Autodesk Inventor part; units mm, degrees
(part 2 of 2)
sketch "Sketch10" plane through (0, 0, 3.75) normal (0, 0, 1) x (1, 0, 0)
  line L0 (-21, 11) -> (-21, -11) projected
  line L1 (-21, -11) -> (-15, -11) projected
  line L2 (-15, -11) -> (-15, 11) projected
  line L3 (-15, 11) -> (-21, 11) projected
  line L4 (-20, 10) -> (-16, 10) projected
  line L5 (-16, 10) -> (-16, -10) projected
  line L6 (-16, -10) -> (-20, -10) projected
  line L7 (-20, -10) -> (-20, 10) projected
  line L8 (6, 21) -> (-6, 21) projected
  line L9 (-6, 21) -> (-6, 15) projected
  line L10 (-6, 15) -> (6, 15) projected
  line L11 (6, 15) -> (6, 21) projected
  line L12 (-5.1733, 20) -> (5.0327, 20) projected
  line L13 (5.0327, 20) -> (5.0327, 16) projected
  line L14 (5.0327, 16) -> (-5.1733, 16) projected
  line L15 (-5.1733, 16) -> (-5.1733, 20) projected
  line L16 (18.5, -10) -> (18.5, 9) projected
  line L17 (18.5, 9) -> (16, 9) projected
  line L18 (16, 9) -> (16, -10) projected
  line L19 (16, -10) -> (18.5, -10) projected
  line L20 (17.6346, -9) -> (16.861, -9) projected
  line L21 (16.861, -9) -> (16.861, -8) projected
  line L22 (16.861, -8) -> (17.6346, -8) projected
  line L23 (17.6346, -8) -> (17.6346, -9) projected
  line L24 (17.6346, -7) -> (16.861, -7) projected
  line L25 (16.861, -7) -> (16.861, -6) projected
  line L26 (16.861, -6) -> (17.6346, -6) projected
  line L27 (17.6346, -6) -> (17.6346, -7) projected
  line L28 (17.6346, -5) -> (16.861, -5) projected
  line L29 (16.861, -5) -> (16.861, -4) projected
  line L30 (16.861, -4) -> (17.6346, -4) projected
  line L31 (17.6346, -4) -> (17.6346, -5) projected
  line L32 (17.6346, -3) -> (16.861, -3) projected
  line L33 (16.861, -3) -> (16.861, -2) projected
  line L34 (16.861, -2) -> (17.6346, -2) projected
  line L35 (17.6346, -2) -> (17.6346, -3) projected
  line L36 (17.6337, -1.0613) -> (16.8602, -1.0613) projected
  line L37 (16.8602, -1.0613) -> (16.8602, -0.0613) projected
  line L38 (16.8602, -0.0613) -> (17.6337, -0.0613) projected
  line L39 (17.6337, -0.0613) -> (17.6337, -1.0613) projected
  line L40 (17.6337, 1.1028) -> (16.8602, 1.1028) projected
  line L41 (16.8602, 1.1028) -> (16.8602, 2.1028) projected
  line L42 (16.8602, 2.1028) -> (17.6337, 2.1028) projected
  line L43 (17.6337, 2.1028) -> (17.6337, 1.1028) projected
  line L44 (17.6346, 3) -> (16.861, 3) projected
  line L45 (16.861, 3) -> (16.861, 4) projected
  line L46 (16.861, 4) -> (17.6346, 4) projected
  line L47 (17.6346, 4) -> (17.6346, 3) projected
  line L48 (17.6346, 5) -> (16.861, 5) projected
  line L49 (16.861, 5) -> (16.861, 6) projected
  line L50 (16.861, 6) -> (17.6346, 6) projected
  line L51 (17.6346, 6) -> (17.6346, 5) projected
  line L52 (16.861, 8) -> (17.6346, 8) projected
  line L53 (17.6346, 8) -> (17.6346, 7) projected
  line L54 (17.6346, 7) -> (16.861, 7) projected
  line L55 (16.861, 7) -> (16.861, 8) projected
  line L56 (-19, -3) -> (-19, -2.5) projected
  line L57 (-19, -2.5) -> (-18.3156, -2.5) projected
  line L58 (-18.3156, -2.5) -> (-18.3156, -3) projected
  line L59 (-18.3156, -3) -> (-19, -3) projected
  line L60 (-19, 1.4327) -> (-19, 1.9327) projected
  line L61 (-19, 1.9327) -> (-18.3156, 1.9327) projected
  line L62 (-18.3156, 1.9327) -> (-18.3156, 1.4327) projected
  line L63 (-18.3156, 1.4327) -> (-19, 1.4327) projected
  line L64 (-19, 8) -> (-19, 8.5) projected
  line L65 (-19, 8.5) -> (-18.3156, 8.5) projected
  line L66 (-18.3156, 8.5) -> (-18.3156, 8) projected
  line L67 (-18.3156, 8) -> (-19, 8) projected
  line L68 (-20, 10) -> (-20, -10) projected
  line L69 (-20, -10) -> (-16, -10) projected
  line L70 (-16, -10) -> (-16, 10) projected
  line L71 (-16, 10) -> (-20, 10) projected
  line L72 (-19, -6) -> (-19, -5.5) projected
  line L73 (-19, -5.5) -> (-18.3156, -5.5) projected
  line L74 (-18.3156, -5.5) -> (-18.3156, -6) projected
  line L75 (-18.3156, -6) -> (-19, -6) projected
  line L76 (-19, 4.8259) -> (-19, 5.3259) projected
  line L77 (-19, 5.3259) -> (-18.3156, 5.3259) projected
  line L78 (-18.3156, 5.3259) -> (-18.3156, 4.8259) projected
  line L79 (-18.3156, 4.8259) -> (-19, 4.8259) projected
  line L80 (-19, -8.4464) -> (-19, -7.9464) projected
  line L81 (-19, -7.9464) -> (-18.3156, -7.9464) projected
  line L82 (-18.3156, -7.9464) -> (-18.3156, -8.4464) projected
  line L83 (-18.3156, -8.4464) -> (-19, -8.4464) projected
  line L84 (-5.1733, 20) -> (-5.1733, 16) projected
  line L85 (-5.1733, 16) -> (5.0327, 16) projected
  line L86 (5.0327, 16) -> (5.0327, 20) projected
  line L87 (5.0327, 20) -> (-5.1733, 20) projected
  line L88 (1.2968, 18.5) -> (1.2968, 19) projected
  line L89 (1.2968, 19) -> (2.1134, 19) projected
  line L90 (2.1134, 19) -> (2.1134, 18.5) projected
  line L91 (2.1134, 18.5) -> (1.2968, 18.5) projected
  line L92 (-4.3467, 18.5) -> (-4.3467, 19) projected
  line L93 (-4.3467, 19) -> (-3.5998, 19) projected
  line L94 (-3.5998, 19) -> (-3.5998, 18.5) projected
  line L95 (-3.5998, 18.5) -> (-4.3467, 18.5) projected
  line L96 (3.6544, 19) -> (4.5488, 19) projected
  line L97 (4.5488, 19) -> (4.5488, 18.5) projected
  line L98 (4.5488, 18.5) -> (3.6544, 18.5) projected
  line L99 (3.6544, 18.5) -> (3.6544, 19) projected
  line L100 (-1.5055, 18.5) -> (-1.5055, 19) projected
  line L101 (-1.5055, 19) -> (-0.7289, 19) projected
  line L102 (-0.7289, 19) -> (-0.7289, 18.5) projected
  line L103 (-0.7289, 18.5) -> (-1.5055, 18.5) projected
  point P0 (0, 0)
extrude "Extrusion10" add sketch "Sketch10" along normal blind 5.5
sketch "Sketch11" plane through (-16, 21, 0) normal (0, 1, 0) x (1, 0, 0)
  line L0 (10, -1.25) -> (10, -9.25) projected
  line L1 (22, -9.25) -> (10, -9.25) projected
  line L2 (22, -1.25) -> (22, -9.25) projected
  line L3 (22, -1.25) -> (22, -9.25) projected
  line L4 (10, -1.25) -> (22, -1.25)
  point P0 (16, 0)
  constraints: 2 end point, 1 perpendicular
extrude "Extrusion11" add sketch "Sketch11" along normal blind 0.005
sketch "Sketch12" plane through (21, -16, 0) normal (1, 0, 0) x (0, 0, -1)
  line L0 (-2.75, 24) -> (-2.75, 7) projected
  line L1 (-1.25, 7) -> (-2.75, 7) projected
  line L2 (-1.25, 24) -> (-2.75, 24) projected
  line L3 (-1.25, 24) -> (-1.25, 7)
  point P0 (0, 16)
  constraints: 2 end point
extrude "Extrusion12" add sketch "Sketch12" along normal blind 0.005
sketch "Sketch13" plane through (-21, -16, 0) normal (-1, 0, 0) x (0, 0, 1)
  line L0 (1.25, 5) -> (9.25, 5) projected
  line L1 (9.25, 27) -> (9.25, 5) projected
  line L2 (1.25, 27) -> (9.25, 27) projected
  line L3 (1.25, 27) -> (1.25, 5) projected
  line L4 (1.25, 27) -> (1.25, 5)
  point P0 (0, 16)
  constraints: 2 end point
extrude "Extrusion13" add sketch "Sketch13" along normal blind 0.005
sketch "Sketch14" plane through (0, 0, 1.25) normal (0, 0, 1) x (1, 0, 0)
  line L0 (6, -8.4464) -> (6, -10) projected
  line L1 (-8, 0) -> (-8, -7) projected
  line L2 (-13, -7) -> (-13, 0) projected
  line L3 (11, 2.5) -> (2.5, 2.5) projected
  line L4 (3.1309, 2.5) -> (4, 2.5)
  line L5 (4, 2.5) -> (4, 2)
  line L6 (4, 2) -> (3.1309, 2)
  line L7 (3.1309, 2) -> (3.1309, 2.5)
  line L8 (5.0085, 2.5) -> (5.8776, 2.5)
  line L9 (5.8776, 2.5) -> (5.8776, 2)
  line L10 (5.8776, 2) -> (5.0085, 2)
  line L11 (5.0085, 2) -> (5.0085, 2.5)
  line L12 (7.1309, 2.5) -> (8, 2.5)
  line L13 (8, 2.5) -> (8, 2)
  line L14 (8, 2) -> (7.1309, 2)
  line L15 (7.1309, 2) -> (7.1309, 2.5)
  line L16 (9.1309, 2.5) -> (10, 2.5)
  line L17 (10, 2.5) -> (10, 2)
  line L18 (10, 2) -> (9.1309, 2)
  line L19 (9.1309, 2) -> (9.1309, 2.5)
  line L20 (3.1309, 5.2581) -> (4, 5.2581)
  line L21 (4, 5.2581) -> (4, 4.7581)
  line L22 (4, 4.7581) -> (3.1309, 4.7581)
  line L23 (3.1309, 4.7581) -> (3.1309, 5.2581)
  line L24 (5.0085, 5.2581) -> (5.8776, 5.2581)
  line L25 (5.8776, 5.2581) -> (5.8776, 4.7581)
  line L26 (5.8776, 4.7581) -> (5.0085, 4.7581)
  line L27 (5.0085, 4.7581) -> (5.0085, 5.2581)
  line L28 (7.1309, 5.2581) -> (8, 5.2581)
  line L29 (8, 5.2581) -> (8, 4.7581)
  line L30 (8, 4.7581) -> (7.1309, 4.7581)
  line L31 (7.1309, 4.7581) -> (7.1309, 5.2581)
  line L32 (9.1309, 5.2581) -> (10, 5.2581)
  line L33 (10, 5.2581) -> (10, 4.7581)
  line L34 (10, 4.7581) -> (9.1309, 4.7581)
  line L35 (9.1309, 4.7581) -> (9.1309, 5.2581)
  line L36 (-13, -6.1309) -> (-13, -7)
  line L37 (-13, -7) -> (-13.5, -7)
  line L38 (-13.5, -7) -> (-13.5, -6.1309)
  line L39 (-13.5, -6.1309) -> (-13, -6.1309)
  line L40 (-13, -4.1309) -> (-13, -5)
  line L41 (-13, -5) -> (-13.5, -5)
  line L42 (-13.5, -5) -> (-13.5, -4.1309)
  line L43 (-13.5, -4.1309) -> (-13, -4.1309)
  line L44 (-13.5, -2.8776) -> (-13.5, -2.0085)
  line L45 (-13, -2.0085) -> (-13, -2.8776)
  line L46 (-13, -2.8776) -> (-13.5, -2.8776)
  line L47 (-13.5, -2.0085) -> (-13, -2.0085)
  line L48 (-13, -0.1309) -> (-13, -1)
  line L49 (-13, -1) -> (-13.5, -1)
  line L50 (-13.5, -1) -> (-13.5, -0.1309)
  line L51 (-13.5, -0.1309) -> (-13, -0.1309)
  line L52 (-14.5, 7.4915) -> (-14, 7.4915)
  line L53 (-7.5, -6.1309) -> (-7.5, -7)
  line L54 (-7.5, -7) -> (-8, -7)
  line L55 (-8, -7) -> (-8, -6.1309)
  line L56 (-8, -6.1309) -> (-7.5, -6.1309)
  line L57 (-7.5, -4.1309) -> (-7.5, -5)
  line L58 (-7.5, -5) -> (-8, -5)
  line L59 (-8, -5) -> (-8, -4.1309)
  line L60 (-8, -4.1309) -> (-7.5, -4.1309)
  line L61 (-8, -2.8776) -> (-8, -2.0085)
  line L62 (-7.5, -2.0085) -> (-7.5, -2.8776)
  line L63 (-7.5, -2.8776) -> (-8, -2.8776)
  line L64 (-8, -2.0085) -> (-7.5, -2.0085)
  line L65 (-7.5, -0.1309) -> (-7.5, -1)
  line L66 (-7.5, -1) -> (-8, -1)
  line L67 (-8, -1) -> (-8, -0.1309)
  line L68 (-8, -0.1309) -> (-7.5, -0.1309)
  line L69 (-14.5, 3.5) -> (-14.5, 4.3691)
  line L70 (-14.5, 4.3691) -> (-14, 4.3691)
  line L71 (-14, 3.5) -> (-14.5, 3.5)
  line L72 (-14, 4.3691) -> (-14, 3.5)
  line L73 (-14, 5.6224) -> (-14.5, 5.6224)
  line L74 (-14, 6.4915) -> (-14, 5.6224)
  line L75 (-14.5, 8.3691) -> (-14, 8.3691)
  line L76 (-14.5, 7.5) -> (-14.5, 8.3691)
  line L77 (-14, 8.3691) -> (-14, 7.5)
  line L78 (-14, 7.5) -> (-14.5, 7.5)
  line L79 (-14.5, 6.4915) -> (-14, 6.4915)
  line L80 (-14.5, 5.6224) -> (-14.5, 6.4915)
  line L81 (-11.9931, 3.557) -> (-11.9931, 4.426)
  line L82 (-11.9931, 4.426) -> (-11.4931, 4.426)
  line L83 (-11.4931, 3.557) -> (-11.9931, 3.557)
  line L84 (-11.4931, 4.426) -> (-11.4931, 3.557)
  line L85 (-11.4931, 5.6794) -> (-11.9931, 5.6794)
  line L86 (-11.4931, 6.5484) -> (-11.4931, 5.6794)
  line L87 (-11.9931, 8.426) -> (-11.4931, 8.426)
  line L88 (-11.9931, 7.557) -> (-11.9931, 8.426)
  line L89 (-11.4931, 8.426) -> (-11.4931, 7.557)
  line L90 (-11.4931, 7.557) -> (-11.9931, 7.557)
  line L91 (-11.9931, 6.5484) -> (-11.4931, 6.5484)
  line L92 (-11.9931, 5.6794) -> (-11.9931, 6.5484)
  line L93 (-14, 4.3691) -> (-14, 3.5)
  line L94 (-14, 8.3691) -> (-14, 7.4915)
  line L95 (-14, 6.4915) -> (-14, 5.6224)
  line L96 (1.713, -11.4558) -> (3.1309, -11.4558) projected
  line L97 (3.1309, -11.4558) -> (3.1309, -7) projected
  line L98 (3.1309, -7) -> (1.713, -7) projected
  line L99 (1.713, -7) -> (1.713, -11.4558) projected
  line L100 (6.25, -11.4558) -> (8, -11.4558) projected
  line L101 (8, -11.4558) -> (8, -7) projected
  line L102 (8, -7) -> (6.25, -7) projected
  line L103 (6.25, -7) -> (6.25, -11.4558) projected
  line L104 (8.5, -10.6055) -> (8, -10.6055)
  line L105 (8, -10.6055) -> (8, -9.7364)
  line L106 (8.5, -9.7364) -> (8.5, -10.6055)
  line L107 (8, -9.7364) -> (8.5, -9.7364)
  line L108 (8, -7.8588) -> (8.5, -7.8588)
  line L109 (8.5, -7.8588) -> (8.5, -8.7279)
  line L110 (8.5, -8.7279) -> (8, -8.7279)
  line L111 (8, -8.7279) -> (8, -7.8588)
  line L112 (3.6309, -10.4337) -> (3.1309, -10.4337)
  line L113 (3.1309, -10.4337) -> (3.1309, -9.5646)
  line L114 (3.6309, -9.5646) -> (3.6309, -10.4337)
  line L115 (3.1309, -9.5646) -> (3.6309, -9.5646)
  line L116 (3.1309, -7.687) -> (3.6309, -7.687)
  line L117 (3.6309, -7.687) -> (3.6309, -8.5561)
  line L118 (3.6309, -8.5561) -> (3.1309, -8.5561)
  line L119 (3.1309, -8.5561) -> (3.1309, -7.687)
  line L120 (1.213, -10.4337) -> (1.713, -10.4337)
  line L121 (1.213, -9.5646) -> (1.213, -10.4337)
  line L122 (1.713, -9.5646) -> (1.213, -9.5646)
  line L123 (1.713, -10.4337) -> (1.713, -9.5646)
  line L124 (1.213, -8.5561) -> (1.713, -8.5561)
  line L125 (1.213, -7.687) -> (1.213, -8.5561)
  line L126 (1.713, -7.687) -> (1.213, -7.687)
  line L127 (1.713, -8.5561) -> (1.713, -7.687)
  line L128 (5.75, -10.6055) -> (6.25, -10.6055)
  line L129 (5.75, -9.7364) -> (5.75, -10.6055)
  line L130 (6.25, -9.7364) -> (5.75, -9.7364)
  line L131 (6.25, -10.6055) -> (6.25, -9.7364)
  line L132 (5.75, -8.7279) -> (6.25, -8.7279)
  line L133 (5.75, -7.8588) -> (5.75, -8.7279)
  line L134 (6.25, -7.8588) -> (5.75, -7.8588)
  line L135 (6.25, -8.7279) -> (6.25, -7.8588)
  point P0 (-13, -3.5)
  point P1 (-8, -3.5)
  point P2 (6, -9.7364)
  point P3 (6, -8.7279)
  constraints: 248 end point, 52 parallel, 26 perpendicular, 8 horizontal, 2 midpoint, 1 point on line
extrude "Extrusion14" add sketch "Sketch14" along normal blind 1 contours L132 L103 L130 L0 | L132 L133 L134 L103 | L130 L103 L128 L129 | L108 L109 L110 L101 | L101 L107 L106 L104 | L68 L65 L66 L1 | L56 L53 L54 L1 | L60 L57 L58 L1 | L64 L62 L63 L1 | L37 L38 L39 L2 | L49 L50 L51 L2 | L46 L44 L47 L2 | L41 L42 L43 L2 | L17 L18 L19 L3 | L5 L6 L7 L3 | L9 L10 L11 L3 | L13 L14 L15 L3 | L20 L21 L22 L23 | L24 L25 L26 L27 | L28 L29 L30 L31 | L32 L33 L34 L35 | L69 L70 L72 L71 | L73 L80 L79 L74 | L75 L77 L78 L76 | L81 L82 L84 L83 | L85 L92 L91 L86 | L87 L89 L90 L88 | L120 L121 L122 L99 | L97 L115 L114 L112 | L124 L125 L126 L99 | L97 L116 L117 L118
sketch "Sketch15" plane through (0, 0, 1.25) normal (0, 0, 1) x (1, 0, 0)
  line L0 (-3, -14.5088) -> (-1.7185, -14.5088)
  line L1 (-1.7185, -14.5088) -> (-1.7185, -15.2453)
  line L2 (-1.7185, -15.2453) -> (-3, -15.2453)
  line L3 (-3, -15.2453) -> (-3, -14.5088)
  line L4 (2.8155, -12.5) -> (0, -12.5)
  line L5 (0, -12.5) -> (0, -14)
  line L6 (0, -14) -> (2.8155, -14)
  line L7 (2.8155, -14) -> (2.8155, -12.5)
  line L8 (0, -15.2453) -> (2.8155, -15.2453)
  line L9 (2.8155, -15.2453) -> (2.8155, -16.25)
  line L10 (2.8155, -16.25) -> (0, -16.25)
  line L11 (0, -16.25) -> (0, -15.2453)
  line L12 (-1, -18) -> (1, -18)
  line L13 (1, -18) -> (1, -20)
  line L14 (1, -20) -> (-1, -20)
  line L15 (-1, -20) -> (-1, -18)
  line L16 (6.7991, -4.25) -> (9.1309, -4.25)
  line L17 (9.1309, -4.25) -> (9.1309, -5)
  line L18 (9.1309, -5) -> (6.7991, -5)
  line L19 (6.7991, -5) -> (6.7991, -4.25)
  line L20 (0, 0) -> (1.4077, 0)
  line L21 (1.4077, 0) -> (1.4077, -1.0613)
  line L22 (1.4077, -1.0613) -> (0, -1.0613)
  line L23 (0, -1.0613) -> (0, 0)
  line L24 (2.422, 0) -> (3.6309, 0)
  line L25 (3.6309, 0) -> (3.6309, -1.0613)
  line L26 (3.6309, -1.0613) -> (2.422, -1.0613)
  line L27 (2.422, -1.0613) -> (2.422, 0)
  line L28 (-1, 0) -> (-2.3592, 0)
  line L29 (-2.3592, 0) -> (-2.3592, -1.0613)
  line L30 (-2.3592, -1.0613) -> (-1, -1.0613)
  line L31 (-1, -1.0613) -> (-1, 0)
  line L32 (6.25, -13.25) -> (7.125, -13.25)
  line L33 (7.125, -13.25) -> (7.125, -14)
  line L34 (7.125, -14) -> (6.25, -14)
  line L35 (6.25, -14) -> (6.25, -13.25)
  line L36 (8.5, -13.25) -> (9.5, -13.25)
  line L37 (9.5, -13.25) -> (9.5, -14)
  line L38 (9.5, -14) -> (8.5, -14)
  line L39 (8.5, -14) -> (8.5, -13.25)
  line L40 (13.3629, 3.9915) -> (14, 3.9915)
  line L41 (14, 3.9915) -> (14, 2)
  line L42 (14, 2) -> (13.3629, 2)
  line L43 (13.3629, 2) -> (13.3629, 3.9915)
  line L44 (13.3629, 0) -> (14, 0)
  line L45 (14, 0) -> (14, -2.0085)
  line L46 (14, -2.0085) -> (13.3629, -2.0085)
  line L47 (13.3629, -2.0085) -> (13.3629, 0)
  line L48 (-11, 17.5088) -> (-9.5, 17.5088)
  line L49 (-9.5, 17.5088) -> (-9.5, 16.5785)
  line L50 (-9.5, 16.5785) -> (-11, 16.5785)
  line L51 (-11, 16.5785) -> (-11, 17.5088)
  line L52 (-11, 15.6095) -> (-9.5, 15.6095)
  line L53 (-9.5, 15.6095) -> (-9.5, 14.5)
  line L54 (-9.5, 14.5) -> (-11, 14.5)
  line L55 (-11, 14.5) -> (-11, 15.6095)
  line L56 (9.5, 16) -> (11, 16)
  line L57 (11, 16) -> (11, 14.7955)
  line L58 (11, 14.7955) -> (9.5, 14.7955)
  line L59 (9.5, 14.7955) -> (9.5, 16)
  constraints: 120 end point, 30 parallel, 17 point on line, 15 horizontal, 15 perpendicular
extrude "Extrusion15" add sketch "Sketch15" along normal blind 0.75
body "Solid1"
